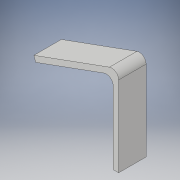
# Autodesk Inventor part: 70DegreeHinge
Saved by Autodesk Inventor 2017 (Build 210142000, 142)
## iProperties
Created: 2017-10-24
Part Number: 70DegreeHinge
Material: Generic
Document SubType Name: Modeling
Designer: Aidan_Moga
Density: 1 g/cm^3
Appearance: Default
Author: Aidan_Moga
Autodesk Inventor part; units mm, degrees
ref_plane "YZ Plane" through (0, 0, 0) normal (1, 0, 0) x (0, 1, 0)
ref_plane "XZ Plane" through (0, 0, 0) normal (0, 1, 0) x (-1, 0, 0)
ref_plane "XY Plane" through (0, 0, 0) normal (0, 0, 1) x (1, 0, 0)
sketch "Sketch1" plane through (0, 0, 0) normal (0, 0, 1) x (1, 0, 0)
  line L0 (0, 0) -> (0, 38.1)
  line L1 (0, 38.1) -> (-35.8023, 25.069)
  line L2 (0, 0) -> (2.54, 0)
  line L3 (2.54, 0) -> (2.54, 41.7275)
  line L4 (-35.8023, 25.069) -> (-36.671, 27.4559)
  line L5 (-36.671, 27.4559) -> (2.54, 41.7275)
  dimension "d0" = 38.1
  dimension "d1" = 38.1
  dimension "d2" = 70
  dimension "d3" = 2.54
  dimension "d4" = 2.54
  constraints: 12 end point, 2 perpendicular, 1 horizontal, 1 vertical
  measures "d0" distance of L0.start L0.end
  measures "d1" distance of L0.end L1.end
  measures "d2" angle of L1 L0
  measures "d3" distance of L0.start L2.end
  measures "d4" distance of L1.end L4.end
extrude "Extrusion1" add sketch "Sketch1" along normal blind 12.7
fillet "Fillet1" radius 3.175 2 edges at (2.54, 41.7275, 6.35) (0, 38.1, 6.35)
body "Solid1"
